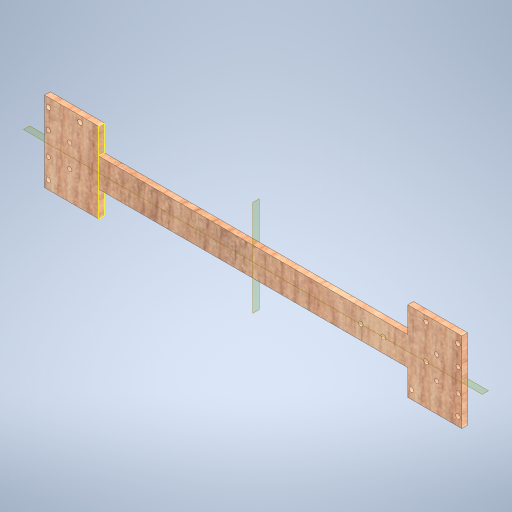
# Autodesk Inventor part: центр_рейка
Saved by Autodesk Inventor 2023.1 (Build 271208000, 208)
## iProperties
Created: 2025-12-22
Part Number: центр_рейка
Material: Древесина (береза)
Document SubType Name: Modeling
Designer: DELL
Density: 0.55 g/cm^3
Appearance: Береза — натуральный — полированный
Author: DELL
Autodesk Inventor part; units mm, degrees
ref_plane "YZ Plane" through (0, 0, 0) normal (1, 0, 0) x (0, 1, 0)
ref_plane "XZ Plane" through (0, 0, 0) normal (0, 1, 0) x (-1, 0, 0)
ref_plane "XY Plane" through (0, 0, 0) normal (0, 0, 1) x (1, 0, 0)
sketch "Эскиз1" plane through (0, 0, 0) normal (0, 0, 1) x (1, 0, 0)
  circle A0 centre (-7.5, -22.95) radius 1.5 projected
  circle A1 centre (7.5, -22.95) radius 1.5 projected
  circle A2 centre (7.5, -6.95) radius 1.5 projected
  circle A3 centre (-7.5, -6.95) radius 1.5 projected
  line L0 (-281.4, 13.05) -> (10, 13.05)
  line L1 (10, 13.05) -> (10, -42.95)
  line L2 (10, -42.95) -> (-281.4, -42.95)
  line L3 (-281.4, -42.95) -> (-281.4, 13.05)
  line L4 (-281.4, 13.05) -> (10, -42.95) construction
  line L5 (10, 13.05) -> (-281.4, -42.95) construction
  line L6 (-135.7, -14.95) -> (-135.7, -42.95) construction
  circle A4 centre (-263.9, -22.95) radius 1.5
  circle A5 centre (-278.9, -22.95) radius 1.5
  circle A6 centre (-278.9, -6.95) radius 1.5
  circle A7 centre (-263.9, -6.95) radius 1.5
  point P0 (0, 0)
  dimension "d5" = 291.4
  dimension "d8" = 2.5
  dimension "d9" = 20
  dimension "d10" = 20
  constraints: 14 end point, 4 centre point, 4 symmetric about line, 3 midpoint, 2 parallel, 1 horizontal, 1 perpendicular, 4 other
  measures "d5" distance of L1.end L2.end
  measures "d8" distance from line of L1 A2.centre
  measures "d9" distance from line of L0 A2.centre
  measures "d10" distance from line of L2 A0.centre
extrude "Выдавливание1" add sketch "Эскиз1" along normal blind 4
sketch "Эскиз4" plane through (0, 0, 0) normal (0, 0, -1) x (-1, 0, 0)
  line L0 (27.7, 31.05) -> (243.7, 31.05)
  line L1 (243.7, 31.05) -> (243.7, -4.95)
  line L2 (243.7, -4.95) -> (27.7, -4.95)
  line L3 (27.7, -4.95) -> (27.7, 31.05)
  line L4 (-10, 13.05) -> (281.4, 13.05) projected
  line L5 (27.7, 31.05) -> (243.7, -4.95) construction
  line L6 (243.7, 31.05) -> (27.7, -4.95) construction
  point P0 (0, 0)
  point P1 (135.7, 13.05)
  point P2 (243.7, 13.05)
  dimension "d13" = 18
  dimension "d14" = 216
  constraints: 12 end point, 4 midpoint, 2 parallel, 1 horizontal, 1 perpendicular
  measures "d13" distance of L1.end point (243.7, 13.05)
  measures "d14" distance of L1.end L2.end
extrude "Выдавливание3" cut sketch "Эскиз4" against normal blind 4
ref_plane "РабПлоскость1" through (-281.4, -14.95, 0) normal (0, -1, 0) x (1, 0, 0)
mirror "Зеркальное отражение1" about plane through (-281.4, -14.95, 0) normal (0, -1, 0) of "Выдавливание3"
sketch "Эскиз8" plane through (0, 0, 4) normal (0, 0, 1) x (1, 0, 0)
  circle A0 centre (-278.8, -36.95) radius 1.6 projected
  line L0 (-243.7, -42.95) -> (-243.7, -24.95) projected
  line L1 (-281.4, -42.95) -> (-243.7, -42.95) projected
  circle A1 centre (-278.8, 7.05) radius 1.6
  point P0 (0, 0)
  dimension "d48" = 3.2
  dimension "d49" = 44
  constraints: 1 centre point
  measures "d48" diameter of A1
  measures "d49" distance of A0.centre A1.centre
extrude "Выдавливание7" cut sketch "Эскиз8" against normal blind 10
ref_plane "РабПлоскость2" through (-135.7, -42.95, 0) normal (-1, 0, 0) x (0, 0, 1)
mirror "Зеркальное отражение2" about plane through (-135.7, -42.95, 0) normal (-1, 0, 0) of "Выдавливание7"
sketch "Эскиз10" plane through (0, 0, 4) normal (0, 0, 1) x (1, 0, 0)
  circle A0 centre (7.4, -36.95) radius 1.6 projected
  circle A1 centre (-25.1, -36.95) radius 1.6
  point P0 (0, 0)
  dimension "d50" = 3.2
  dimension "d51" = 32.5
  constraints: 1 centre point
  measures "d50" diameter of A1
  measures "d51" distance of A0.centre A1.centre
extrude "Выдавливание8" cut sketch "Эскиз10" against normal blind 10
sketch "Эскиз11" plane through (0, 0, 4) normal (0, 0, 1) x (1, 0, 0)
  circle A0 centre (-256.6, 9.05) radius 1.6 projected
  point P0 (0, 0)
extrude "Выдавливание9" cut sketch "Эскиз11" against normal blind 10
mirror "Зеркальное отражение4" about plane through (-135.7, -42.95, 0) normal (-1, 0, 0) of "Выдавливание9"
sketch "Эскиз12" plane through (0, 0, 4) normal (0, 0, 1) x (1, 0, 0)
  circle A0 centre (-14.8, -14.95) radius 1.6
  line L0 (-243.7, -24.95) -> (-27.7, -24.95) projected
  circle A1 centre (-14.8, 9.05) radius 1.6 projected
  line L1 (-14.8, -24.95) -> (-14.8, 9.05) construction
  circle A2 centre (-60.5, -14.95) radius 1.6
  circle A3 centre (-44.8, -14.95) radius 1.6 projected
  point P0 (0, 0)
  dimension "d56" = 3.2
  dimension "d57" = 10
  dimension "d58" = 3.2
  dimension "d59" = 45.7
  constraints: 2 centre point, 2 end point, 1 point on line, 1 vertical
  measures "d56" diameter of A0
  measures "d57" distance from line of L0 A0.centre
  measures "d58" diameter of A2
  measures "d59" distance of A0.centre A2.centre
extrude "Выдавливание10" cut sketch "Эскиз12" against normal blind 10 contours A0 | A2 | A3
sketch "Эскиз14" plane through (-243.7, -42.95, 0) normal (1, 0, 0) x (0, 0, -1)
  line L0 (0, 56) -> (0, 38) projected
  line L1 (0, 38) -> (0, 18) projected
  line L2 (0, 18) -> (-4, 18) projected
  line L3 (-4, 0) -> (-4, 18) projected
  line L4 (0, 0) -> (-4, 0) projected
  line L5 (0, 18) -> (0, 0) projected
  line L6 (-4, 56) -> (0, 56) projected
  line L7 (-4, 38) -> (-4, 56) projected
  line L8 (-4, 38) -> (0, 38) projected
  line L9 (-4, 18) -> (-4, 38) projected
  point P0 (0, 42.95)
